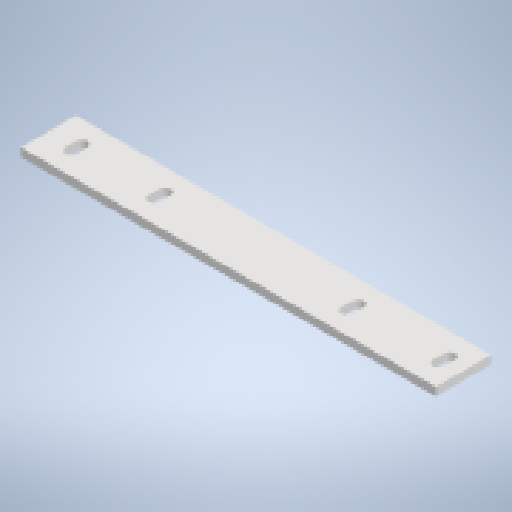
# Autodesk Inventor part: 발받침대위,아래
Saved by Autodesk Inventor 2024 (Build 280153000, 153)
## iProperties
Created: 2024-04-09
Part Number: 발받침대위,아래
Material: 일반
Document SubType Name: Modeling
Designer: ckhye
Density: 1 g/cm^3
Appearance: 기본값
Author: ckhye
Autodesk Inventor part; units mm, degrees
ref_plane "YZ Plane" through (0, 0, 0) normal (1, 0, 0) x (0, 1, 0)
ref_plane "XZ Plane" through (0, 0, 0) normal (0, 1, 0) x (-1, 0, 0)
ref_plane "XY Plane" through (0, 0, 0) normal (0, 0, 1) x (1, 0, 0)
sketch "스케치1" plane through (0, 0, 0) normal (0, 1, 0) x (-1, 0, 0)
  line L0 (75, 10) -> (-75, 10)
  line L1 (-75, 10) -> (-75, -10)
  line L2 (-75, -10) -> (75, -10)
  line L3 (75, -10) -> (75, 10)
  line L4 (75, 10) -> (-75, -10) construction
  line L5 (-75, 10) -> (75, -10) construction
  circle A0 centre (35, 0) radius 2.25
  line L6 (105, 0) -> (-105, 0) projected
  circle A1 centre (-35, 0) radius 2.25
  point P0 (0, 0)
  point P1 (-75, 0)
  dimension "d0" = 150
  dimension "d1" = 20
  dimension "d4" = 4.5
  dimension "d5" = 40
  dimension "d6" = 4.5
  dimension "d7" = 40
  constraints: 12 end point, 3 midpoint, 2 centre point, 2 parallel, 2 point on line, 1 horizontal, 1 perpendicular
  measures "d0" distance of L2.end L1.end
  measures "d1" distance between parallel lines of L2 L0
  measures "d4" diameter of A0
  measures "d5" distance from line of L3 A0.centre
  measures "d6" diameter of A1
  measures "d7" distance of point (-75, 0) A1.centre
extrude "돌출1" add sketch "스케치1" along normal blind 3
sketch "스케치4" plane through (0, 0, 0) normal (0, -1, 0) x (1, 0, 0)
  line L0 (-35, -2) -> (-35, 2) construction
  line L1 (-33, -2) -> (-33, 2)
  line L2 (-37, 2) -> (-37, -2)
  arc A0 (-37, -2) -> (-33, -2) centre (-35, -2) ccw
  arc A1 (-33, 2) -> (-37, 2) centre (-35, 2) ccw
  line L3 (35, -2) -> (35, 2) construction
  line L4 (37, -2) -> (37, 2)
  line L5 (33, 2) -> (33, -2)
  arc A2 (33, -2) -> (37, -2) centre (35, -2) ccw
  arc A3 (37, 2) -> (33, 2) centre (35, 2) ccw
  line L6 (-75, 10) -> (75, 10) projected
  line L7 (75, 10) -> (75, -10) projected
  line L8 (-75, -10) -> (-75, 10) projected
  line L9 (75, -10) -> (-75, -10) projected
  line L10 (68, 2) -> (68, -2) construction
  line L11 (66, 2) -> (66, -2)
  line L12 (70, -2) -> (70, 2)
  arc A4 (70, 2) -> (66, 2) centre (68, 2) ccw
  arc A5 (66, -2) -> (70, -2) centre (68, -2) ccw
  line L13 (-65, -2) -> (-65, 2) construction
  line L14 (-63, -2) -> (-63, 2)
  line L15 (-67, 2) -> (-67, -2)
  arc A6 (-67, -2) -> (-63, -2) centre (-65, -2) ccw
  arc A7 (-63, 2) -> (-67, 2) centre (-65, 2) ccw
  point P0 (-35, 0)
  point P1 (35, 0)
  point P2 (68, 0)
  point P3 (-65, 0)
  point P4 (75, 0)
  point P5 (75, 0)
  point P6 (-75, 0)
  point P7 (-75, 0)
  dimension "d14" = 4
  dimension "d15" = 4
  dimension "d16" = 4
  dimension "d17" = 4
  dimension "d18" = 10
  dimension "d19" = 40
  dimension "d20" = 10
  dimension "d21" = 40
  dimension "d28" = 4
  dimension "d29" = 4
  dimension "d30" = 4
  dimension "d31" = 4
  dimension "d32" = 0
  dimension "d33" = 7
  dimension "d34" = 0
  dimension "d35" = 10
  constraints: 32 end point, 16 point on circle, 16 tangent, 8 centre point, 8 midpoint, 6 parallel, 1 perpendicular, 1 vertical
  measures "d14" distance of L0.start L0.end
  measures "d15" diameter of A1
  measures "d16" distance of L3.start L3.end
  measures "d17" diameter of A3
  measures "d18" distance from line of L6 point (35, 0)
  measures "d19" distance from line of L7 point (35, 0)
  measures "d20" distance from line of L6 point (-35, 0)
  measures "d21" distance from line of L8 point (-35, 0)
  measures "d28" distance of L10.start L10.end
  measures "d29" diameter of A5
  measures "d30" distance of L13.start L13.end
  measures "d31" diameter of A7
  measures "d32" vertical distance of point (75, 0) point (68, 0)
  measures "d33" distance of point (75, 0) point (68, 0)
  measures "d34" vertical distance of point (-75, 0) point (-65, 0)
  measures "d35" distance of point (-75, 0) point (-65, 0)
extrude "돌출3" cut sketch "스케치4" against normal blind 10 contours A0 L2 A1 L1 | A2 L5 A3 L4 | A4 L12 A5 L11 | A6 L15 A7 L14
